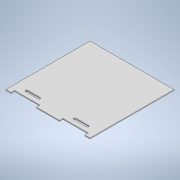
# Autodesk Inventor part: FreePanel
Saved by Autodesk Inventor 2020 (Build 240168000, 168)
## iProperties
Created: 2021-11-12
Part Number: FreePanel
Material: Generic
Document SubType Name: Sheet Metal
Designer: 17185
Density: 1 g/cm^3
Sheet Metal Rule: Default
Appearance: Default
Author: 17185
Autodesk Inventor part; units mm, degrees
ref_plane "YZ Plane" through (0, 0, 0) normal (1, 0, 0) x (0, 1, 0)
ref_plane "XZ Plane" through (0, 0, 0) normal (0, 1, 0) x (-1, 0, 0)
ref_plane "XY Plane" through (0, 0, 0) normal (0, 0, 1) x (1, 0, 0)
sketch "Sketch1" plane through (0, 0, 0) normal (0, 1, 0) x (-1, 0, 0)
  line L0 (152.4, 152.4) -> (-152.4, 152.4)
  line L1 (-152.4, 152.4) -> (-152.4, -152.4)
  line L2 (-152.4, -152.4) -> (152.4, -152.4)
  line L3 (152.4, -152.4) -> (152.4, 152.4)
  line L4 (152.4, 152.4) -> (-152.4, -152.4) construction
  line L5 (-152.4, 152.4) -> (152.4, -152.4) construction
  point P0 (0, 0)
  dimension "d0" = 304.8
  dimension "d1" = 304.8
  measures "d0" distance of L1.end L2.end
  measures "d1" distance of L2.end L0.start
extrude "Plate1" add sketch "Sketch1" along normal blind 3.048
sketch "Sketch2" plane through (0, 3.048, 0) normal (0, 1, 0) x (1, 0, 0)
  line L0 (-152.4, -152.4) -> (152.4, -152.4) projected
  line L1 (-133.35, -139.7) -> (-41.91, -139.7)
  line L2 (-41.91, -139.7) -> (-41.91, -165.1)
  line L3 (-41.91, -165.1) -> (-133.35, -165.1)
  line L4 (-133.35, -165.1) -> (-133.35, -139.7)
  line L5 (-133.35, -139.7) -> (-41.91, -165.1) construction
  line L6 (-41.91, -139.7) -> (-133.35, -165.1) construction
  line L7 (41.91, -139.7) -> (133.35, -139.7)
  line L8 (133.35, -139.7) -> (133.35, -165.1)
  line L9 (133.35, -165.1) -> (41.91, -165.1)
  line L10 (41.91, -165.1) -> (41.91, -139.7)
  line L11 (41.91, -139.7) -> (133.35, -165.1) construction
  line L12 (133.35, -139.7) -> (41.91, -165.1) construction
  line L13 (-152.4, -152.4) -> (-152.4, 152.4) projected
  line L14 (152.4, 152.4) -> (152.4, -152.4) projected
  point P0 (0, 0)
  point P1 (-87.63, -152.4)
  point P2 (87.63, -152.4)
  dimension "d7" = 91.44
  dimension "d8" = 25.4
  dimension "d9" = 91.44
  dimension "d10" = 25.4
  dimension "d11" = 19.05
  dimension "d12" = 19.05
  constraints: 24 end point, 4 midpoint, 4 parallel, 2 horizontal, 2 perpendicular, 2 point on line
  measures "d7" distance of L2.end L3.end
  measures "d8" distance of L1.end L2.end
  measures "d9" distance of L8.end L9.end
  measures "d10" distance of L7.end L8.end
  measures "d11" distance between parallel lines of L13 L4
  measures "d12" distance between parallel lines of L8 L14
extrude "Cut1" cut sketch "Sketch2" against normal blind 3.048
sketch "Sketch3" plane through (0, 3.048, 0) normal (0, 1, 0) x (1, 0, 0)
  line L0 (-110.49, -119.888) -> (-64.77, -119.888) construction
  line L1 (-110.49, -116.078) -> (-64.77, -116.078)
  line L2 (-64.77, -123.698) -> (-110.49, -123.698)
  arc A0 (-110.49, -116.078) -> (-110.49, -123.698) centre (-110.49, -119.888) ccw
  arc A1 (-64.77, -123.698) -> (-64.77, -116.078) centre (-64.77, -119.888) ccw
  line L3 (-152.4, -152.4) -> (-152.4, 152.4) projected
  line L4 (-133.35, -139.7) -> (-41.91, -139.7) projected
  line L5 (-41.91, -152.4) -> (41.91, -152.4) construction
  line L6 (0, -152.4) -> (0, 0) construction
  line L7 (110.49, -119.888) -> (64.77, -119.888) construction
  line L8 (110.49, -116.078) -> (64.77, -116.078)
  line L9 (64.77, -123.698) -> (110.49, -123.698)
  arc A2 (110.49, -123.698) -> (110.49, -116.078) centre (110.49, -119.888) ccw
  arc A3 (64.77, -116.078) -> (64.77, -123.698) centre (64.77, -119.888) ccw
  point P0 (-87.63, -119.888)
  point P1 (87.63, -119.888)
  dimension "d13" = 41.91
  dimension "d14" = 45.72
  dimension "d15" = 3.81
  dimension "d16" = 19.812
  constraints: 18 end point, 8 point on circle, 7 symmetric about line, 4 centre point, 4 tangent, 2 midpoint, 1 horizontal, 1 parallel, 1 vertical, 2 other
  measures "d13" distance from line of L3 L0.start
  measures "d14" distance of L0.start L0.end
  measures "d15" radius of A1
  measures "d16" distance from line of L4 point (-87.63, -119.888)
extrude "Cut2" cut sketch "Sketch3" against normal blind 3.048
equation "\"d5\" = Thickness"
equation "\"d17\" = Thickness"
equation "\"d2\" = Thickness"
equation "\"BendRadius\" = Thickness"
equation "\"BendReliefWidth\" = Thickness"
equation "\"BendReliefDepth\" = 0.5 * Thickness"
equation "\"CornerReliefSize\" = 4 * Thickness"
equation "\"MinimumRemnant\" = 2 * Thickness"
equation "\"TransitionRadius\" = BendRadius"
equation "\"JacobiRadiusSize\" = BendRadius"
equation "\"GapSize\" = Thickness"
equation "\"Thickness\" = 3.048"
body "Solid1"
